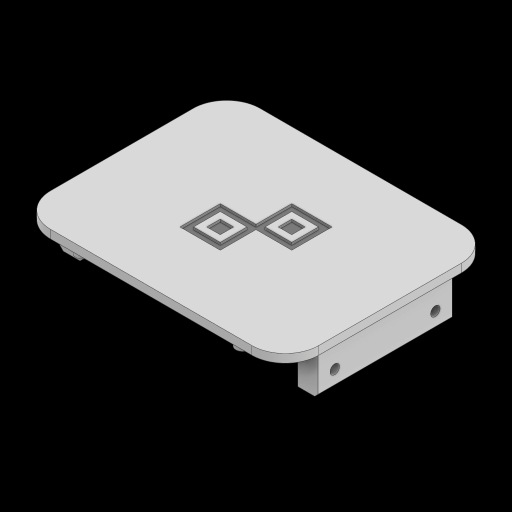
# Autodesk Inventor part: 240_Backplate
Saved by Autodesk Inventor 2024 (Build 280153000, 153)
## iProperties
Created: 2023-07-20
Part Number: 240_Backplate
Material: Generisch
Document SubType Name: Modeling
Designer: Philipp
Density: 1 g/cm^3
Appearance: Vorgabe
Author: Philipp
Autodesk Inventor part; units mm, degrees
ref_plane "YZ Plane" through (0, 0, 0) normal (1, 0, 0) x (0, 1, 0)
ref_plane "XZ Plane" through (0, 0, 0) normal (0, 1, 0) x (-1, 0, 0)
ref_plane "XY Plane" through (0, 0, 0) normal (0, 0, 1) x (1, 0, 0)
sketch "Skizze1" plane through (0, 0, 0) normal (0, 0, 1) x (1, 0, 0)
  line L0 (-80, 62.5) -> (80, 62.5)
  line L1 (80, 62.5) -> (80, -62.5)
  line L2 (80, -62.5) -> (-80, -62.5)
  line L3 (-80, -62.5) -> (-80, 62.5)
  line L4 (-80, 62.5) -> (80, -62.5) construction
  line L5 (80, 62.5) -> (-80, -62.5) construction
  point P0 (0, 0)
  dimension "d0" = 160
  dimension "d1" = 125
  constraints: 12 end point, 2 midpoint, 2 parallel, 1 horizontal, 1 perpendicular
  measures "d0" distance of L1.end L2.end
  measures "d1" distance of L0.end L1.end
extrude "Extrusion1" add sketch "Skizze1" along normal blind 5
fillet "Rundung1" radius 20 4 edges at (80, 62.5, 2.5) (80, -62.5, 2.5) (-80, -62.5, 2.5) (-80, 62.5, 2.5)
sketch "Skizze2" plane through (0, 0, 5) normal (0, 0, 1) x (1, 0, 0)
  line L0 (6.6667, 14.6667) -> (14.6667, 14.6667)
  line L1 (14.6667, 14.6667) -> (14.6667, 6.6667)
  line L2 (14.6667, 6.6667) -> (6.6667, 6.6667)
  line L3 (6.6667, 6.6667) -> (6.6667, 14.6667)
  line L4 (6.6667, 14.6667) -> (14.6667, 6.6667) construction
  line L5 (14.6667, 14.6667) -> (6.6667, 6.6667) construction
  line L6 (2.6667, 18.6667) -> (18.6667, 18.6667)
  line L7 (18.6667, 18.6667) -> (18.6667, 2.6667)
  line L8 (18.6667, 2.6667) -> (2.6667, 2.6667)
  line L9 (2.6667, 2.6667) -> (2.6667, 18.6667)
  line L10 (2.6667, 18.6667) -> (18.6667, 2.6667) construction
  line L11 (18.6667, 18.6667) -> (2.6667, 2.6667) construction
  line L12 (-1.3333, 22.6667) -> (22.6667, 22.6667)
  line L13 (22.6667, 22.6667) -> (22.6667, -1.3333)
  line L14 (22.6667, -1.3333) -> (-1.3333, -1.3333)
  line L15 (-1.3333, -1.3333) -> (-1.3333, 22.6667)
  line L16 (-1.3333, 22.6667) -> (22.6667, -1.3333) construction
  line L17 (22.6667, 22.6667) -> (-1.3333, -1.3333) construction
  line L18 (-10.6667, -10.6667) -> (10.6667, -10.6667) construction
  line L19 (10.6667, -10.6667) -> (10.6667, 10.6667) construction
  line L20 (10.6667, 10.6667) -> (-10.6667, 10.6667) construction
  line L21 (-10.6667, 10.6667) -> (-10.6667, -10.6667) construction
  line L22 (-10.6667, -10.6667) -> (10.6667, 10.6667) construction
  line L23 (10.6667, -10.6667) -> (-10.6667, 10.6667) construction
  line L24 (60, 62.5) -> (-60, 62.5) construction
  line L25 (80, -42.5) -> (80, 42.5) construction
  line L26 (-14.6667, -14.6667) -> (-14.6667, -6.6667)
  line L27 (-14.6667, -6.6667) -> (-6.6667, -6.6667)
  line L28 (-6.6667, -6.6667) -> (-6.6667, -14.6667)
  line L29 (-6.6667, -14.6667) -> (-14.6667, -14.6667)
  line L30 (-6.6667, -6.6667) -> (-14.6667, -14.6667) construction
  line L31 (-2.6667, -2.6667) -> (-2.6667, -18.6667)
  line L32 (-18.6667, -2.6667) -> (-2.6667, -2.6667)
  line L33 (-18.6667, -18.6667) -> (-18.6667, -2.6667)
  line L34 (-2.6667, -18.6667) -> (-18.6667, -18.6667)
  line L35 (-2.6667, -2.6667) -> (-18.6667, -18.6667) construction
  line L36 (-18.6667, -2.6667) -> (-2.6667, -18.6667) construction
  line L37 (1.3333, -22.6667) -> (-22.6667, -22.6667)
  line L38 (-22.6667, 1.3333) -> (1.3333, 1.3333)
  line L39 (-22.6667, -22.6667) -> (-22.6667, 1.3333)
  line L40 (1.3333, 1.3333) -> (1.3333, -22.6667)
  line L41 (-22.6667, 1.3333) -> (1.3333, -22.6667) construction
  line L42 (1.3333, 1.3333) -> (-22.6667, -22.6667) construction
  line L43 (-14.6667, -6.6667) -> (-6.6667, -14.6667) construction
  point P0 (0, 0)
  point P1 (1.3333, -1.3333)
  point P2 (-1.3333, 1.3333)
  dimension "d14" = 8
  dimension "d15" = 8
  dimension "d16" = 16
  dimension "d17" = 16
  dimension "d18" = 24
  dimension "d20" = 21.3333
  dimension "d21" = 21.3333
  dimension "d22" = 62.5
  dimension "d23" = 80
  dimension "d24" = 8
  dimension "d25" = 8
  dimension "d26" = 16
  dimension "d27" = 16
  dimension "d28" = 24
  constraints: 84 end point, 14 midpoint, 14 parallel, 7 horizontal, 7 perpendicular, 2 point on line
  measures "d14" distance of L3.end L0.end
  measures "d15" distance of L0.end L1.end
  measures "d16" distance of L6.start L7.start
  measures "d17" distance of L7.start L7.end
  measures "d18" distance of L12.end L14.start
  measures "d20" distance of L19.end L20.end
  measures "d21" distance of L18.end L19.end
  measures "d22" distance from line of L24 point (0, 0)
  measures "d23" distance from line of L25 point (0, 0)
  measures "d24" distance of L26.end L28.start
  measures "d25" distance of L28.start L29.start
  measures "d26" distance of L32.start L32.end
  measures "d27" distance of L32.end L31.end
  measures "d28" distance of L40.start L37.start
extrude "Extrusion2" cut sketch "Skizze2" against normal blind 1.5
sketch "Skizze3" plane through (0, 0, 0) normal (0, 0, -1) x (-1, 0, 0)
  circle A0 centre (50, -53.5) radius 4
  line L0 (60, -62.5) -> (-60, -62.5) projected
  line L1 (80, 42.5) -> (80, -42.5) projected
  line L2 (50, -53.5) -> (-45.5, -53.5)
  line L3 (-45.5, -53.5) -> (-45.5, 25)
  line L4 (-45.5, 25) -> (50, 25)
  line L5 (50, 25) -> (50, -53.5)
  circle A1 centre (-45.5, -53.5) radius 4
  circle A2 centre (-45.5, 25) radius 4
  circle A3 centre (50, 25) radius 4
  circle A4 centre (-45.5, 25) radius 2
  circle A5 centre (50, 25) radius 2
  circle A6 centre (50, -53.5) radius 2
  circle A7 centre (-45.5, -53.5) radius 2
  point P0 (0, 0)
  dimension "d31" = 9
  dimension "d32" = 30
  dimension "d33" = 8
  dimension "d34" = 78.5
  dimension "d35" = 95.5
  dimension "d36" = 8
  dimension "d37" = 8
  dimension "d38" = 8
  dimension "d39" = 4
  dimension "d40" = 4
  dimension "d41" = 4
  dimension "d42" = 4
  constraints: 8 centre point, 8 end point, 7 coincident, 2 parallel, 1 horizontal, 1 perpendicular
  measures "d31" distance from line of L0 L2.start
  measures "d32" distance from line of L1 L2.start
  measures "d33" diameter of A0
  measures "d34" distance of L2.end L3.end
  measures "d35" distance of L3.end L4.end
  measures "d36" diameter of A1
  measures "d37" diameter of A2
  measures "d38" diameter of A3
  measures "d39" diameter of A4
  measures "d40" diameter of A5
  measures "d41" diameter of A6
  measures "d42" diameter of A7
extrude "Extrusion3" add sketch "Skizze3" along normal blind 7 contours A0 L2 A6 L5 | L5 A6 L2 A0 | A3 L4 A5 L5 | L5 A5 L4 A3 | A1 L3 A7 L2 | L2 A7 L3 A1 | A2 L3 A4 L4 | L4 A4 L3 A2
sketch "Skizze4" plane through (0, 0, 0) normal (0, 0, -1) x (-1, 0, 0)
  line L0 (-80, -42.5) -> (-80, 42.5) projected
  line L1 (80, 42.5) -> (80, -42.5) projected
  line L2 (-77, 40) -> (-65, 40)
  line L3 (-65, 40) -> (-65, -40)
  line L4 (-65, -40) -> (-77, -40)
  line L5 (-77, -40) -> (-77, 40)
  line L6 (77, 40) -> (65, 40)
  line L7 (65, 40) -> (65, -40)
  line L8 (65, -40) -> (77, -40)
  line L9 (77, -40) -> (77, 40)
  point P0 (0, 0)
  point P1 (-71, 40)
  dimension "d45" = 3
  dimension "d46" = 80
  dimension "d47" = 40
  dimension "d48" = 12
  dimension "d49" = 3
  dimension "d50" = 12
  dimension "d51" = 80
  dimension "d52" = 40
  constraints: 16 end point, 4 parallel, 2 horizontal, 2 perpendicular, 1 midpoint
  measures "d45" distance between parallel lines of L0 L5
  measures "d46" distance of L2.end L3.end
  measures "d47" vertical distance of point (0, 0) point (-71, 40)
  measures "d48" distance of L2.start L2.end
  measures "d49" distance between parallel lines of L1 L9
  measures "d50" distance of L6.start L6.end
  measures "d51" distance of L6.end L7.end
  measures "d52" distance from line of point (0, 0) L6
extrude "Extrusion4" add sketch "Skizze4" along normal blind 25
sketch "Skizze5" plane through (77, -40, 0) normal (1, 0, 0) x (0, 0, -1)
  line L0 (0, 0) -> (0, 80) projected
  line L1 (0, 0) -> (25, 0) projected
  line L2 (25, 80) -> (25, 0) projected
  line L3 (0, 80) -> (25, 80) projected
  line L4 (0, -2.5) -> (0, 82.5) projected
  point P0 (0, 40)
  point P1 (15, 70)
  point P2 (15, 10)
  point P3 (0, 40)
  point P4 (0, 40)
  dimension "d55" = 30
  dimension "d56" = 30
  dimension "d57" = 15
  dimension "d58" = 15
  constraints: 2 midpoint
  measures "d55" vertical distance of point (0, 40) point (15, 70)
  measures "d56" vertical distance of point (0, 40) point (15, 10)
  measures "d57" distance from line of L0 point (15, 10)
  measures "d58" distance from line of L0 point (15, 70)
hole "Bohrung1" at (77, 30, -15) at (77, -30, -15) direction (-1, 0, 0) diameter 5.6 depth 154 tip angle 118
chamfer "Fasen1" distance 2 angle 45 2 edges at (77, 0, -25) (-77, 0, -25)
equation "\"d14\" = d24"
equation "\"d15\" = d14"
equation "\"d16\" = 2 * d14"
equation "\"d17\" = d16"
equation "\"d18\" = 3 * d14"
equation "\"d20\" = 2.66667 * d24"
equation "\"d21\" = d20"
equation "\"d25\" = d24"
equation "\"d26\" = 2 * d24"
equation "\"d27\" = d26"
equation "\"d28\" = 3 * d24"
equation "\"d47\" = 0.5 * d46"
equation "\"d52\" = 0.5 * d51"
